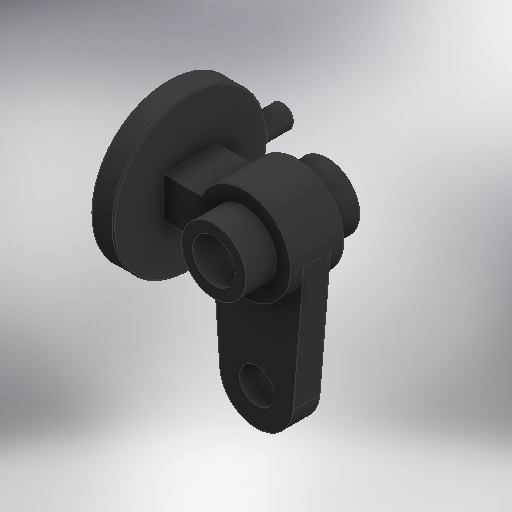
# Autodesk Inventor part: travainterna
Saved by Autodesk Inventor 2025.3 (Build 293356000, 356)
## iProperties
Created: 2026-09-18
Part Number: travainterna
Material: Genérico
Document SubType Name: Modeling
Designer: user
Density: 1 g/cm^3
Appearance: Padrão
Author: user
Autodesk Inventor part; units mm, degrees
ref_plane "YZ Plane" through (0, 0, 0) normal (1, 0, 0) x (0, 1, 0)
ref_plane "XZ Plane" through (0, 0, 0) normal (0, 1, 0) x (-1, 0, 0)
sketch "Esboço1" plane through (0, 0, 0) normal (0, 0, 1) x (1, 0, 0)
  circle A0 centre (0, 0) radius 3.5
  circle A1 centre (0, 0) radius 1.6
  dimension "d0" = 7
  dimension "d1" = 3.2
  constraints: 2 centre point, 2 coincident
  measures "d0" diameter of A0
  measures "d1" diameter of A1
extrude "Extrusão1" add sketch "Esboço1" along normal blind 4
ref_plane "Plano de trabalho1" through (0, 0, 2) normal (0, 0, 1) x (1, 0, 0)
sketch "Esboço2" plane through (0, 0, 2) normal (0, 0, 1) x (1, 0, 0)
  circle A0 centre (0, 0) radius 1.6
  circle A1 centre (0, 0) radius 2.425
  dimension "d5" = 4.85
  dimension "d37" = 3.2
  constraints: 2 centre point, 2 coincident
  measures "d5" diameter of A1
  measures "d37" diameter of A0
extrude "Extrusão2" add sketch "Esboço2" along normal blind 4.25 and the other way blind 4.25
sketch "Esboço3" plane through (0, 0, 2) normal (0, 0, 1) x (1, 0, 0)
  circle A0 centre (-0.0504, -9.7495) radius 2.75
  circle A1 centre (-0.0504, -9.7495) radius 1.3
  circle A2 centre (0, 0) radius 3.5 projected
  circle A3 centre (0, 0) radius 3.5 projected
  line L0 (0, -7) -> (0, -3.5)
  line L1 (2.6903, -9.9753) -> (3.4882, -0.2873)
  line L2 (-2.7933, -9.9469) -> (-3.491, -0.2512)
  line L3 (-0.0504, -12.4995) -> (-7.6035, -15.5853)
  line L4 (0, 3.5) -> (-11.1989, 6.8937)
  point P0 (-3.491, -0.2512)
  point P1 (3.4882, -0.2873)
  dimension "d15" = 3.5
  dimension "d38" = 2.6
  constraints: 10 end point, 8 point on circle, 4 tangent, 2 centre point, 1 coincident
  measures "d15" distance of L0.start L0.end
  measures "d38" diameter of A1
extrude "Extrusão3" add sketch "Esboço3" along normal blind 1 and the other way blind 1 contours A0 | A0 L0 A2 L1 | A0 L2 A2 L0
sketch "Esboço4" plane through (0, 0, 2) normal (0, 0, 1) x (1, 0, 0)
  circle A0 centre (0, 0) radius 3.5 projected
  line L0 (-3.1623, 1.5) -> (-6, 1.5)
  line L1 (-6, 1.5) -> (-6, -1.5)
  line L2 (-6, -1.5) -> (-3.1623, -1.5)
  constraints: 6 end point, 2 point on circle, 1 horizontal, 1 parallel, 1 perpendicular
extrude "Extrusão4" add sketch "Esboço4" along normal blind 2 and the other way blind 2 contours A0 L2 L1 L0
sketch "Esboço5" plane through (-6, -1.5, 4) normal (-1, 0, 0) x (0, 0, 1)
  line L0 (-2, 1.5) -> (4.2682, 3.8776) construction
  circle A0 centre (-2, 1.5) radius 5.775
  point P0 (-4, 1.5)
  dimension "d29" = 11.55
  constraints: 2 end point, 1 centre point, 1 coincident
  measures "d29" diameter of A0
extrude "Extrusão5" add sketch "Esboço5" along normal blind 1.7
sketch "Esboço6" plane through (0, 0, 2) normal (0, 0, 1) x (1, 0, 0)
  line L0 (-6, -1.5) -> (-6, 1.5) projected
  line L1 (-6, 0) -> (-7.7, 0)
  line L2 (-7.7, 5.775) -> (-7.7, -5.775) projected
  circle A0 centre (-6.85, 0) radius 0.85
  point P0 (0, 0)
  constraints: 3 midpoint, 2 end point, 1 horizontal alignment, 2 other
extrude "Extrusão6" add sketch "Esboço6" against normal blind 7.8
fillet "Arredondamento2" radius 0.1 5 edges at (-7.7, 5.775, 2) (-7.7, -5.775, 2) (-6, 5.775, 2) (-6, -5.775, 2) (-7.7, 0, -5.8)
